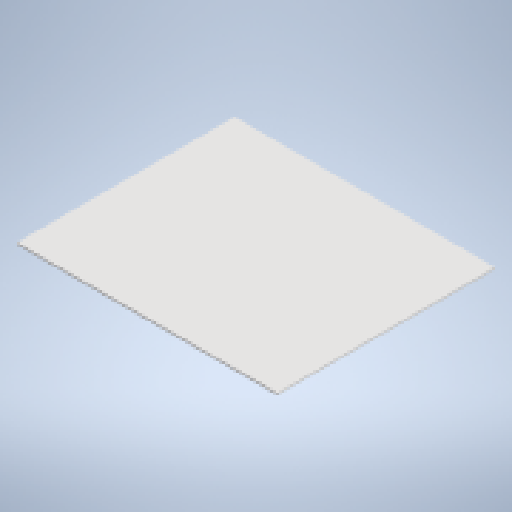
# Autodesk Inventor part: Base
Saved by Autodesk Inventor 2024 (Build 280153000, 153)
## iProperties
Created: 2023-07-06
Part Number: Base
Material: Generic
Document SubType Name: Modeling
Designer: Gabriel Marquez
Density: 1 g/cm^3
Appearance: Default
Author: Gabriel Marquez
Autodesk Inventor part; units mm, degrees
ref_plane "YZ Plane" through (0, 0, 0) normal (1, 0, 0) x (0, 1, 0)
ref_plane "XZ Plane" through (0, 0, 0) normal (0, 1, 0) x (-1, 0, 0)
ref_plane "XY Plane" through (0, 0, 0) normal (0, 0, 1) x (1, 0, 0)
sketch "Sketch1" plane through (0, 0, 0) normal (0, 1, 0) x (-1, 0, 0)
  line L0 (0, 0) -> (820.42, 0)
  line L1 (820.42, 0) -> (820.42, 685.8)
  line L2 (820.42, 685.8) -> (0, 685.8)
  line L3 (0, 685.8) -> (0, 0)
  dimension "d0" = 820.42
  dimension "d1" = 685.8
  constraints: 8 end point, 2 parallel, 1 horizontal, 1 perpendicular
  measures "d0" distance of L2.end L1.end
  measures "d1" distance of L1.end L0.end
extrude "Extrusion1" add sketch "Sketch1" along normal blind 6.35
body "Solid1"
